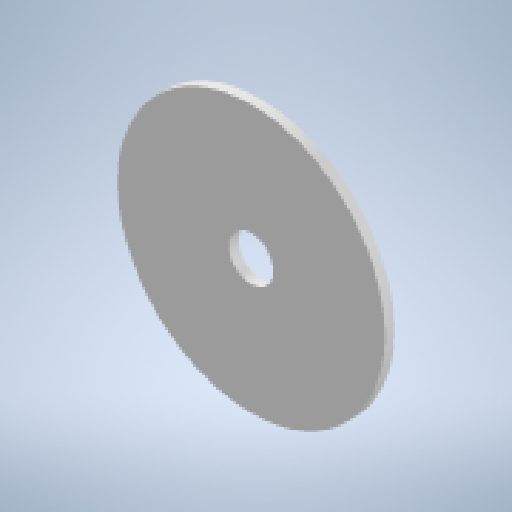
# Autodesk Inventor part: BaseTopPlate
Saved by Autodesk Inventor 2023 (Build 270158030, 158C)
## iProperties
Created: 2024-10-14
Part Number: BaseTopPlate
Material: Generic
Document SubType Name: Modeling
Designer: lvrectanus0
Density: 1 g/cm^3
Appearance: Default
Author: lvrectanus0
Autodesk Inventor part; units mm, degrees
ref_plane "YZ Plane" through (0, 0, 0) normal (1, 0, 0) x (0, 1, 0)
ref_plane "XZ Plane" through (0, 0, 0) normal (0, 1, 0) x (-1, 0, 0)
ref_plane "XY Plane" through (0, 0, 0) normal (0, 0, 1) x (1, 0, 0)
sketch "Sketch1" plane through (0, 0, 0) normal (0, 0, 1) x (1, 0, 0)
  circle A0 centre (0, 0) radius 14.2875 projected
  circle A1 centre (0, 0) radius 86.1483 projected
  point P0 (0, 0)
ref_plane "Work Plane1" through (-15.4305, -15.4305, -6.096) normal (0, 0, 1) x (1, 0, 0)
extrude "Extrusion1" add sketch "Sketch1" against normal up to surface (6.096 mm away)
sketch "Sketch2" plane through (0, 0, 0) normal (0, 0, 1) x (1, 0, 0)
  arc A0 (0.0676, -63.21) -> (-0.0676, -63.21) centre (0, -60.96) ccw projected
  circle A1 centre (0, -60.96) radius 3.175
  point P0 (0, 0)
  dimension "d2" = 6.35
  constraints: 1 centre point, 1 coincident
  measures "d2" diameter of A1
extrude "Extrusion2" cut sketch "Sketch2" against normal through all
chamfer "Chamfer1" distance 1 angle 45 2 edges at (-3.175, -60.96, -6.096) (-3.175, -60.96, 0)
sketch "Sketch3" plane through (0, 0, 0) normal (0, 0, 1) x (1, 0, 0)
  circle A0 centre (0, -60.96) radius 4.175 projected
  line L0 (15.5, -76.46) -> (-15.5, -45.46) construction
  line L1 (15.5, -45.46) -> (-15.5, -76.46) construction
  circle A1 centre (15.5, -76.46) radius 4
  circle A2 centre (-15.5, -76.46) radius 4
  circle A3 centre (-15.5, -45.46) radius 4
  circle A4 centre (15.5, -45.46) radius 4
  point P0 (0, 0)
  dimension "d8" = 31
  dimension "d9" = 31
  dimension "d10" = 8
  constraints: 4 centre point, 4 coincident, 4 end point, 3 equal radius, 2 horizontal alignment, 2 midpoint, 2 vertical alignment
  measures "d8" distance of L1.end L0.start
  measures "d9" distance of L0.end L1.end
  measures "d10" diameter of A1
sketch "Sketch4" plane through (0, 0, 0) normal (0, 0, 1) x (1, 0, 0)
  circle A0 centre (0, 0) radius 86.1483 projected
  circle A1 centre (0, -60.96) radius 3.175 projected
  circle A2 centre (50, 78.74) radius 2
  circle A3 centre (50, 27.94) radius 3
  circle A4 centre (50, 78.74) radius 7.1254
  circle A5 centre (0, 0) radius 86.1483 projected
  arc A6 (25.5581, 82.2698) -> (46.2963, 84.8272) centre (33.0936, 106.5263) ccw
  arc A7 (57.0844, 77.9767) -> (63.5895, 58.1198) centre (82.3382, 75.2559) ccw
  line L0 (0, 0) -> (0, 86.1483) construction
  circle A8 centre (-50, 78.74) radius 2
  circle A9 centre (-50, 27.94) radius 3
  circle A10 centre (-50, 78.74) radius 7.1254
  arc A11 (-46.2963, 84.8272) -> (-25.5581, 82.2698) centre (-33.0936, 106.5263) ccw
  arc A12 (-63.5895, 58.1198) -> (-57.0844, 77.9767) centre (-82.3382, 75.2559) ccw
  point P0 (0, 0)
  dimension "d25" = 60.96
  dimension "d36" = 4
  dimension "d37" = 6
  dimension "d38" = 50.8
  dimension "d39" = 50
  dimension "d40" = 27.94
  dimension "d42" = 25.4
  dimension "d43" = 25.4
  constraints: 15 point on circle, 10 centre point, 8 symmetric about line, 5 tangent, 2 end point, 1 vertical, 1 vertical alignment, 5 other
  measures "d25" distance of A1.centre point (0, 0)
  measures "d36" diameter of A2
  measures "d37" diameter of A3
  measures "d38" distance of A3.centre A2.centre
  measures "d39" horizontal distance of point (0, 0) A3.centre
  measures "d40" vertical distance of A3.centre point (0, 0)
  measures "d42" radius of A6
  measures "d43" radius of A7
extrude "Extrusion3" add sketch "Sketch3" along normal blind 5.08 contours A1 | A2 | A3 | A4
chamfer "Chamfer2" distance 1 angle 45 4 edges at (11.5, -45.46, 0) (11.5, -76.46, 0) (-19.5, -76.46, 0) (-19.5, -45.46, 0)
sketch "Sketch5" plane through (15.5, -76.46, 5.08) normal (0, 0, 1) x (1, 0, 0)
  circle A0 centre (0, 0) radius 4 projected
  circle A1 centre (-31, 0) radius 4 projected
  circle A2 centre (-31, 31) radius 4 projected
  circle A3 centre (0, 31) radius 4 projected
  point P0 (-15.5, 76.46)
hole "Hole1" at (15.5, -76.46, 5.08) at (-15.5, -76.46, 5.08) at (-15.5, -45.46, 5.08) at (15.5, -45.46, 5.08) direction (0, 0, -1) diameter 3.5 end through all
extrude "Extrusion4" add sketch "Sketch4" against normal up to surface (6.096 mm away) contours A0 A4 A7 | A12 A10 A0 | A0 A6 A4 | A4 | A10 A11 A0 | A10 | A2 | A8
hole "Hole2" at (-50, 78.74, 0) at (-50, 27.94, 0) at (50, 27.94, 0) at (50, 78.74, 0) direction (0, 0, -1) diameter 4 end through all
sketch "Sketch6" plane through (0, 0, 0) normal (0, 0, 1) x (1, 0, 0)
  line L0 (0, 0) -> (0, -12.7) construction
  line L1 (31.75, -12.7) -> (81.75, -12.7)
  line L2 (81.75, -12.7) -> (81.75, -6.35)
  line L3 (81.75, -6.35) -> (31.75, -6.35)
  line L4 (31.75, -6.35) -> (31.75, -12.7)
  dimension "d53" = 12.7
  dimension "d54" = 50
  dimension "d55" = 6.35
  dimension "d56" = 31.75
  constraints: 10 end point, 2 parallel, 1 horizontal, 1 horizontal alignment, 1 perpendicular, 1 vertical
  measures "d53" distance of L0.start L0.end
  measures "d54" distance of L3.end L2.end
  measures "d55" distance of L2.end L1.end
  measures "d56" horizontal distance of L0.start L3.end
extrude "Extrusion5" add sketch "Sketch6" along normal blind 50
fillet "Fillet1" radius 10 2 edges at (31.75, -9.525, 50) (81.75, -9.525, 50)
sketch "Sketch7" plane through (41.75, -12.7, 50) normal (0, -1, 0) x (1, 0, 0)
  line L0 (-0.5, -9.5) -> (30.5, -9.5)
  line L1 (30.5, -9.5) -> (30.5, -40.5)
  line L2 (30.5, -40.5) -> (-0.5, -40.5)
  line L3 (-0.5, -40.5) -> (-0.5, -9.5)
  arc A0 (40, -10) -> (30, 0) centre (30, -10) ccw construction
  arc A1 (0, 0) -> (-10, -10) centre (0, -10) ccw construction
  line L4 (30.5, -9.5) -> (-0.5, -40.5) construction
  line L5 (30.5, -40.5) -> (-0.5, -9.5) construction
  point P0 (-41.75, -50)
  point P1 (15, -25)
  point P2 (15, -25)
  dimension "d63" = 31
  dimension "d64" = 31
  constraints: 12 end point, 2 parallel, 2 point on line, 1 coincident, 1 horizontal, 1 midpoint, 1 perpendicular
  measures "d63" distance of L0.start L0.end
  measures "d64" distance of L0.end L1.end
hole "Hole3" at (41.75, -12.7, 40) at (72.25, -12.7, 40.5) at (41.25, -12.7, 9.5) at (72.25, -12.7, 9.5) direction (0, 1, 0) diameter 3.5 end through all
hole "Hole4" at (56.75, -12.7, 25) direction (0, 1, 0) diameter 6 end through all
sketch "Sketch8" plane through (31.75, -6.35, 0) normal (0, 1, 0) x (1, 0, 0)
  line L0 (0, 0) -> (0, -40) projected
  line L1 (0, 0) -> (2.54, 0)
  line L2 (2.54, 0) -> (2.54, -12.7)
  line L3 (2.54, -12.7) -> (0, -12.7)
  line L4 (0, -12.7) -> (0, 0)
  line L5 (50, 0) -> (0, 0) projected
  line L6 (25, 0) -> (22.46, 0)
  line L7 (22.46, 0) -> (22.46, -12.7)
  line L8 (22.46, -12.7) -> (25, -12.7)
  line L9 (25, -12.7) -> (25, 0)
  line L10 (50, 0) -> (47.46, 0)
  line L11 (47.46, 0) -> (47.46, -12.7)
  line L12 (47.46, -12.7) -> (50, -12.7)
  line L13 (50, -12.7) -> (50, 0)
  line L14 (25, 0) -> (27.54, 0)
  line L15 (27.54, 0) -> (27.54, -12.7)
  line L16 (27.54, -12.7) -> (25, -12.7)
  point P0 (-31.75, 0)
  point P1 (22.46, 0)
  dimension "d79" = 2.54
  dimension "d80" = 12.7
  dimension "d81" = 2.54
  dimension "d82" = 12.7
  constraints: 30 end point, 5 symmetric about line, 4 parallel, 2 horizontal, 2 perpendicular, 1 midpoint
  measures "d79" distance of L2.end L3.end
  measures "d80" distance of L1.end L2.end
  measures "d81" distance of L8.end L7.end
  measures "d82" distance of L7.end L6.end
extrude "Extrusion6" add sketch "Sketch8" along normal blind 12.7
chamfer "Chamfer4" distance 12.7 angle 45 3 edges at (80.48, 6.35, 12.7) (56.75, 6.35, 12.7) (33.02, 6.35, 12.7)
chamfer "Chamfer5" distance 3 angle 45 14 edges at (69.25, -6.35, 0) (44.25, -6.35, 0) (31.75, 6.35, 0) (31.75, -3.175, 0) (79.21, 0, 0) (79.21, 6.35, 0) (59.29, 0, 0) (59.29, 6.35, 0) (34.29, 6.35, 0) (34.29, 0, 0) (54.21, 0, 0) (54.21, 6.35, 0) (81.75, -3.175, 0) (81.75, 6.35, 0)
chamfer "Chamfer6" distance 1 angle 45 2 edges at (56.75, -12.7, 28) (56.75, -6.35, 28)
sketch "Sketch9" plane through (0, 0, -6.096) normal (0, 0, -1) x (-1, 0, 0)
  circle A0 centre (15.5, -76.46) radius 1.75 projected
  circle A1 centre (15.5, -45.46) radius 1.75 projected
  circle A2 centre (-15.5, -45.46) radius 1.75 projected
  circle A3 centre (-15.5, -76.46) radius 1.75 projected
  point P0 (0, 0)
  constraints: 4 coincident
hole "Hole5" at (-15.5, -76.46, -6.096) at (-15.5, -45.46, -6.096) at (15.5, -45.46, -6.096) at (15.5, -76.46, -6.096) direction (0, 0, 1) diameter 5 depth 4 tip angle 118
sketch "Sketch10" plane through (41.75, -6.35, 50) normal (0, 1, 0) x (1, 0, 0)
  circle A0 centre (0, 10) radius 1.75 projected
  circle A1 centre (-0.5, 40.5) radius 1.75 projected
  circle A2 centre (30.5, 40.5) radius 1.75 projected
  circle A3 centre (30.5, 9.5) radius 1.75 projected
  point P0 (-41.75, 50)
  constraints: 4 coincident
hole "Hole6" at (41.75, -6.35, 40) at (41.25, -6.35, 9.5) at (72.25, -6.35, 9.5) at (72.25, -6.35, 40.5) direction (0, -1, 0) diameter 5 depth 4 tip angle 118
sketch "Sketch11" plane through (0, 0, 0) normal (0, 0, 1) x (1, 0, 0)
  line L0 (-46.9642, -58.16) -> (-46.9642, -32.76)
  line L1 (-46.9642, -32.76) -> (-34.2642, -32.76)
  line L2 (-34.2642, -32.76) -> (-34.2642, -58.16)
  line L3 (-34.2642, -58.16) -> (-46.9642, -58.16)
  line L4 (-46.9642, -58.16) -> (-34.2642, -32.76) construction
  line L5 (-46.9642, -32.76) -> (-34.2642, -58.16) construction
  line L6 (-46.9642, -58.16) -> (-21.5642, -58.16) construction
  circle A0 centre (0, -60.96) radius 4.175 projected
  circle A1 centre (0, 0) radius 60.96
  circle A2 centre (-15.5, -45.46) radius 5 projected
  line L7 (-46.9642, -45.46) -> (-40.6142, -45.46)
  line L8 (-46.9642, -45.46) -> (-46.9642, -42.92)
  line L9 (-46.9642, -42.92) -> (-44.4242, -42.92)
  line L10 (-44.4242, -42.92) -> (-44.4242, -40.38)
  line L11 (-44.4242, -40.38) -> (-36.8042, -40.38)
  line L12 (-36.8042, -40.38) -> (-36.8042, -50.54)
  line L13 (-36.8042, -50.54) -> (-44.4242, -50.54)
  line L14 (-44.4242, -50.54) -> (-44.4242, -48)
  line L15 (-44.4242, -48) -> (-46.9642, -48)
  line L16 (-46.9642, -45.46) -> (-46.9642, -48)
  point P0 (-40.6142, -45.46)
  point P1 (-40.6142, -45.46)
  dimension "d108" = 25.4
  dimension "d109" = 90
  dimension "d110" = 12.7
  dimension "d111" = 2.54
  dimension "d112" = 2.54
  dimension "d113" = 2.54
  dimension "d114" = 7.62
  dimension "d115" = 10.16
  dimension "d116" = 7.62
  dimension "d117" = 2.54
  constraints: 34 end point, 8 perpendicular, 5 midpoint, 4 point on line, 2 parallel, 2 point on circle, 1 centre point, 1 coincident, 1 horizontal, 1 horizontal alignment
  measures "d108" distance of L0.start L0.end
  measures "d109" angle of L6 L0
  measures "d110" distance of L0.end L1.end
  measures "d111" distance of L7.start L8.end
  measures "d112" distance of L8.end L9.end
  measures "d113" distance of L9.end L10.end
  measures "d114" distance of L10.end L11.end
  measures "d115" distance of L11.end L12.end
  measures "d116" distance of L12.end L13.end
  measures "d117" distance of L13.end L14.end
extrude "Extrusion7" add sketch "Sketch11" along normal up to surface (50 mm away) contours L0 L15 L14 L13 L12 A1 L2 L3 | A1 L12 L11 L10 L0 L1 L2 | L0 A1 L10 L9
chamfer "Chamfer7" distance 1 angle 45 7 edges at (-40.6142, -40.38, 50) (-36.8042, -45.46, 50) (-40.6142, -50.54, 50) (-44.4242, -49.27, 50) (-44.4242, -41.65, 50) (-45.6942, -48, 50) (-45.6942, -42.92, 50)
chamfer "Chamfer8" distance 3 angle 45 3 edges at (-40.6142, -58.16, 0) (-34.2642, -45.46, 0) (-40.6142, -32.76, 0)
sketch "Sketch12" plane through (-46.9642, -58.16, 50) normal (0, -1, 0) x (1, 0, 0)
  line L0 (6.35, -6.35) -> (6.35, -38.1) construction
  line L1 (4.6, -6.35) -> (4.6, -38.1)
  line L2 (8.1, -38.1) -> (8.1, -6.35)
  arc A0 (8.1, -6.35) -> (4.6, -6.35) centre (6.35, -6.35) ccw
  arc A1 (4.6, -38.1) -> (8.1, -38.1) centre (6.35, -38.1) ccw
  line L3 (0, 0) -> (12.7, 0) construction
  line L4 (12.7, 0) -> (0, -12.7) construction
  line L5 (0, -50) -> (0, -1) construction
  line L6 (12.7, 0) -> (30.6605, 0) construction
  line L7 (0, 0) -> (12.7, -12.7) construction
  line L8 (12.7, -47) -> (12.7, 0) construction
  point P0 (46.9642, -50)
  point P1 (6.35, -22.225)
  dimension "d126" = 31.75
  dimension "d127" = 3.5
  dimension "d128" = 135
  constraints: 14 end point, 4 point on circle, 4 tangent, 2 centre point, 2 midpoint, 2 point on line, 1 equal length, 1 horizontal, 1 parallel, 1 vertical
  measures "d126" distance of L0.start L0.end
  measures "d127" diameter of A1
  measures "d128" angle of L4 L6
extrude "Extrusion8" cut sketch "Sketch12" against normal through all
chamfer "Chamfer9" distance 1 angle 45 23 edges at (-46.9642, -32.76, 26.5) (-34.2642, -32.76, 26.5) (-34.2642, -58.16, 26.5) (-46.9642, -58.16, 26.5) (-40.6142, -32.76, 50) (-34.2642, -45.46, 50) (-40.6142, -58.16, 50) (-40.6142, -58.16, 10.15) (-42.3642, -58.16, 27.775) (-40.6142, -58.16, 45.4) (-38.8642, -58.16, 27.775) (-40.6142, -32.76, 45.4) (-42.3642, -32.76, 27.775) (-40.6142, -32.76, 10.15) (-38.8642, -32.76, 27.775) (-40.6142, -40.38, 10.15) (-42.3642, -40.38, 27.775) (-40.6142, -40.38, 45.4) (-38.8642, -40.38, 27.775) (-40.6142, -50.54, 10.15) (-38.8642, -50.54, 27.775) (-40.6142, -50.54, 45.4) (-42.3642, -50.54, 27.775)
sketch "Sketch13" plane through (0, 0, 0) normal (0, 0, 1) x (1, 0, 0)
  circle A0 centre (50, 27.94) radius 2 projected
  circle A1 centre (-50, 78.74) radius 2 projected
  circle A2 centre (-50, 27.94) radius 2 projected
  circle A3 centre (50, 78.74) radius 2 projected
  circle A4 centre (-15.5, -76.46) radius 5 projected
  circle A5 centre (15.5, -45.46) radius 5 projected
  circle A6 centre (0, 0) radius 14.2875 projected
  arc A7 (-63.5895, 58.1198) -> (63.5895, 58.1198) centre (0, 0) ccw projected
  arc A8 (57.0844, 77.9767) -> (63.5895, 58.1198) centre (82.3382, 75.2559) ccw projected
  arc A9 (57.0844, 77.9767) -> (46.2963, 84.8272) centre (50, 78.74) ccw projected
  arc A10 (25.5581, 82.2698) -> (46.2963, 84.8272) centre (33.0936, 106.5263) ccw projected
  arc A11 (25.5581, 82.2698) -> (-25.5581, 82.2698) centre (0, 0) ccw projected
  arc A12 (-46.2963, 84.8272) -> (-25.5581, 82.2698) centre (-33.0936, 106.5263) ccw projected
  arc A13 (-46.2963, 84.8272) -> (-57.0844, 77.9767) centre (-50, 78.74) ccw projected
  arc A14 (-63.5895, 58.1198) -> (-57.0844, 77.9767) centre (-82.3382, 75.2559) ccw projected
  circle A15 centre (0, -60.96) radius 4.175 projected
  circle A16 centre (15.5, -76.46) radius 5 projected
  circle A17 centre (-15.5, -45.46) radius 5 projected
  line L0 (84.75, -12.7) -> (28.75, -12.7) projected
  line L1 (28.75, 6.35) -> (28.75, -12.7) projected
  line L2 (28.75, 6.35) -> (37.29, 6.35) projected
  line L3 (37.29, -3.35) -> (37.29, 6.35) projected
  line L4 (51.21, -3.35) -> (37.29, -3.35) projected
  line L5 (51.21, 6.35) -> (51.21, -3.35) projected
  line L6 (51.21, 6.35) -> (62.29, 6.35) projected
  line L7 (62.29, -3.35) -> (62.29, 6.35) projected
  line L8 (76.21, -3.35) -> (62.29, -3.35) projected
  line L9 (76.21, 6.35) -> (76.21, -3.35) projected
  line L10 (76.21, 6.35) -> (84.75, 6.35) projected
  line L11 (84.75, -12.7) -> (84.75, 6.35) projected
  line L12 (-46.9642, -42.92) -> (-46.9642, -29.76) projected
  line L13 (-31.2642, -29.76) -> (-46.9642, -29.76) projected
  line L14 (-31.2642, -61.16) -> (-31.2642, -29.76) projected
  line L15 (-46.9642, -61.16) -> (-31.2642, -61.16) projected
  line L16 (-46.9642, -61.16) -> (-46.9642, -48) projected
  line L17 (-46.9642, -48) -> (-44.4242, -48) projected
  line L18 (-44.4242, -48) -> (-44.4242, -50.54) projected
  line L19 (-44.4242, -50.54) -> (-36.8042, -50.54) projected
  line L20 (-36.8042, -50.54) -> (-36.8042, -40.38) projected
  line L21 (-36.8042, -40.38) -> (-44.4242, -40.38) projected
  line L22 (-44.4242, -40.38) -> (-44.4242, -42.92) projected
  line L23 (-44.4242, -42.92) -> (-46.9642, -42.92) projected
  circle A18 centre (0, 0) radius 19.3675
  circle A19 centre (-50, 27.94) radius 7.08
  circle A20 centre (50, 27.94) radius 7.08
  line L24 (39.195, 11.43) -> (26.845, 11.43)
  line L25 (23.67, 8.255) -> (23.67, -14.605)
  line L26 (26.845, -17.78) -> (89.83, -17.78)
  line L27 (89.83, -17.78) -> (89.83, 11.43)
  line L28 (76.5119, 11.43) -> (74.305, 11.43)
  line L29 (71.13, 8.255) -> (71.13, 1.73)
  line L30 (71.13, 1.73) -> (67.37, 1.73)
  line L31 (67.37, 1.73) -> (67.37, 8.255)
  line L32 (64.195, 11.43) -> (49.305, 11.43)
  line L33 (46.13, 8.255) -> (46.13, 1.73)
  line L34 (46.13, 1.73) -> (42.37, 1.73)
  line L35 (42.37, 1.73) -> (42.37, 8.255)
  circle A21 centre (15.5, -45.46) radius 10.08
  circle A22 centre (-15.5, -45.46) radius 10.08
  circle A23 centre (0, -60.96) radius 9.255
  circle A24 centre (-15.5, -76.46) radius 10.08
  circle A25 centre (15.5, -76.46) radius 10.08
  line L36 (-29.3592, -24.68) -> (-48.8692, -24.68)
  line L37 (-52.0442, -27.855) -> (-52.0442, -48)
  line L38 (-52.0442, -48) -> (-39.3442, -48)
  line L39 (-39.3442, -48) -> (-39.3442, -45.46)
  line L40 (-39.3442, -45.46) -> (-39.3442, -42.92)
  line L41 (-39.3442, -42.92) -> (-52.0442, -42.92)
  line L42 (-52.0442, -42.92) -> (-52.0442, -66.24)
  line L43 (-52.0442, -66.24) -> (-29.3592, -66.24)
  line L44 (-26.1842, -63.065) -> (-26.1842, -27.855)
  circle A26 centre (-50, 78.74) radius 7.08
  circle A27 centre (50, 78.74) radius 7.08
  arc A28 (79.6306, 15.2003) -> (59.8397, 54.6926) centre (0, 0) ccw
  arc A29 (-59.8397, 54.6926) -> (-52.0336, 78.5209) centre (-82.3382, 75.2559) ccw
  arc A30 (-48.9368, 80.4874) -> (-52.0336, 78.5209) centre (-50, 78.74) ccw
  arc A31 (-48.9368, 80.4874) -> (-24.051, 77.4185) centre (-33.0936, 106.5263) ccw
  arc A32 (24.051, 77.4185) -> (-24.051, 77.4185) centre (0, 0) ccw
  arc A33 (24.051, 77.4185) -> (48.9368, 80.4874) centre (33.0936, 106.5263) ccw
  arc A34 (52.0336, 78.5209) -> (48.9368, 80.4874) centre (50, 78.74) ccw
  arc A35 (52.0336, 78.5209) -> (59.8397, 54.6926) centre (82.3382, 75.2559) ccw
  line L45 (-19.6546, -48.242) -> (-7.6901, -66.1095)
  line L46 (-12.718, -41.3054) -> (5.1495, -53.2699)
  line L47 (12.718, -41.3054) -> (-5.1495, -53.2699)
  line L48 (19.6546, -48.242) -> (7.6901, -66.1095)
  line L49 (19.6546, -73.678) -> (7.6901, -55.8105)
  line L50 (-12.718, -80.6146) -> (5.1495, -68.6501)
  line L51 (-19.6546, -73.678) -> (-7.6901, -55.8105)
  line L52 (12.718, -80.6146) -> (-5.1495, -68.6501)
  line L53 (-20.4324, -44.6406) -> (-25.4437, -74.8082)
  line L54 (-25.4437, -47.1118) -> (-20.4324, -77.2794)
  line L55 (20.4324, -77.2794) -> (25.4437, -47.1118)
  line L56 (20.4324, -44.6406) -> (25.4437, -74.8082)
  line L57 (-16.3194, -40.5276) -> (13.8482, -35.5163)
  line L58 (16.3194, -40.5276) -> (-13.8482, -35.5163)
  circle A36 centre (-50, 78.74) radius 2 projected
  line L59 (-49.0942, 80.5231) -> (50.9058, 29.7231)
  circle A37 centre (50, 27.94) radius 2 projected
  line L60 (49.0942, 26.1569) -> (-50.9058, 76.9569)
  circle A38 centre (-50, 27.94) radius 2 projected
  line L61 (-50.9058, 29.7231) -> (49.0942, 80.5231)
  circle A39 centre (50, 78.74) radius 2 projected
  line L62 (-49.0942, 26.1569) -> (50.9058, 76.9569)
  circle A40 centre (-50, 27.94) radius 2
  circle A41 centre (50, 78.74) radius 2
  circle A42 centre (50, 27.94) radius 2
  circle A43 centre (-50, 78.74) radius 2
  arc A44 (48.0344, 21.1383) -> (-48.0344, 21.1383) centre (0, -145.0737) ccw
  arc A45 (56.0591, 75.0776) -> (56.0591, 31.6024) centre (92.0221, 53.34) ccw
  arc A46 (49.4447, 26.0186) -> (-49.4447, 26.0186) centre (0, -145.0737) ccw
  arc A47 (51.7116, 77.7054) -> (51.7116, 28.9746) centre (92.0221, 53.34) ccw
  arc A48 (-56.0591, 31.6024) -> (-56.0591, 75.0776) centre (-92.0221, 53.34) ccw
  arc A49 (-51.7116, 28.9746) -> (-51.7116, 77.7054) centre (-92.0221, 53.34) ccw
  arc A50 (-45.9629, 33.7562) -> (0, 19.3675) centre (0, 99.9732) ccw
  arc A51 (-19.3675, 0) -> (-47.9379, 21.1669) centre (-41.4937, 0) ccw
  arc A52 (0, 19.3675) -> (45.9629, 33.7562) centre (0, 99.9732) ccw
  arc A53 (47.9379, 21.1669) -> (19.3675, 0) centre (41.4937, 0) ccw
  arc A54 (26.845, 11.43) -> (23.67, 8.255) centre (26.845, 8.255) ccw
  arc A55 (42.37, 8.255) -> (39.195, 11.43) centre (39.195, 8.255) ccw
  arc A56 (49.305, 11.43) -> (46.13, 8.255) centre (49.305, 8.255) ccw
  arc A57 (67.37, 8.255) -> (64.195, 11.43) centre (64.195, 8.255) ccw
  arc A58 (74.305, 11.43) -> (71.13, 8.255) centre (74.305, 8.255) ccw
  arc A59 (76.5119, 11.43) -> (79.6306, 15.2003) centre (76.5119, 14.605) ccw
  arc A60 (23.67, -14.605) -> (26.845, -17.78) centre (26.845, -14.605) ccw
  arc A61 (-63.5895, 58.1198) -> (63.5895, 58.1198) centre (0, 0) ccw projected
  circle A62 centre (0, 0) radius 81.0683
  circle A63 centre (-86.1483, 0) radius 14.2875
  arc A64 (-80.0333, 12.9128) -> (-6.115, 12.9128) centre (-43.0742, 90.9578) ccw
  circle A65 centre (0, 0) radius 14.2875 projected
  arc A66 (-6.115, -12.9128) -> (-80.0333, -12.9128) centre (-43.0742, -90.9578) ccw
  arc A67 (-48.0344, 21.1383) -> (-72.3431, -3.6807) centre (-38.2336, -12.7748) ccw
  arc A68 (-86.3236, 14.2864) -> (-56.0591, 31.6024) centre (-86.7639, 50.1617) ccw
  circle A69 centre (86.1483, 0) radius 14.2875
  arc A70 (6.115, 12.9128) -> (80.0333, 12.9128) centre (43.0742, 90.9578) ccw
  arc A71 (80.0333, -12.9128) -> (10.0594, -16.5502) centre (48.4218, -79.6655) ccw
  arc A72 (-24.4083, -40.7432) -> (-14.2875, 0) centre (-101.3575, 0) ccw
  arc A73 (14.2875, 0) -> (24.4083, -40.7432) centre (101.3575, 0) ccw
  arc A74 (-48.8692, -24.68) -> (-52.0442, -27.855) centre (-48.8692, -27.855) ccw
  arc A75 (-26.1842, -27.855) -> (-29.3592, -24.68) centre (-29.3592, -27.855) ccw
  arc A76 (-29.3592, -66.24) -> (-26.1842, -63.065) centre (-29.3592, -63.065) ccw
  arc A77 (-39.1142, -24.68) -> (-14.2875, 0) centre (-39.1142, 0.1471) ccw
  arc A78 (-65.7994, -47.3552) -> (-52.0442, -42.92) centre (-59.6368, -42.92) ccw
  arc A79 (58.3375, -17.78) -> (25.5003, -46.725) centre (58.3375, -50.8789) ccw
  arc A80 (25.5003, -46.725) -> (52.891, -61.4379) centre (42.0244, -48.8153) ccw
  arc A81 (70.9696, -39.1841) -> (58.3375, -17.78) centre (58.3375, -32.2096) ccw
  arc A82 (72.3431, -3.6807) -> (48.0344, 21.1383) centre (38.2336, -12.7748) ccw
  arc A83 (56.0591, 31.6024) -> (86.3236, 14.2864) centre (86.7639, 50.1617) ccw
  point P0 (0, 0)
  point P1 (0, 27.94)
  point P2 (50, 53.34)
  point P3 (-50, 53.34)
  point P4 (23.1433, -60.96)
  point P5 (21.8667, -53.2748)
  point P6 (14.7847, -55.5146)
  point P7 (11.1383, -60.96)
  point P8 (14.7847, -66.4054)
  point P9 (21.8667, -68.6452)
  point P10 (-6.4091, -80.8146)
  point P11 (6.4091, -80.8146)
  point P12 (5.4454, -75.7447)
  point P13 (0, -72.0983)
  point P14 (-5.4454, -75.7447)
  point P15 (-23.1433, -60.96)
  point P16 (-21.8667, -68.6452)
  point P17 (-14.7847, -66.4054)
  point P18 (-11.1383, -60.96)
  point P19 (-14.7847, -55.5146)
  point P20 (-21.8667, -53.2748)
  point P21 (7.6852, -39.0933)
  point P22 (0, -37.8167)
  point P23 (-7.6852, -39.0933)
  point P24 (-5.4454, -46.1753)
  point P25 (0, -49.8217)
  point P26 (5.4454, -46.1753)
  point P27 (-16.5111, -10.1235)
  point P28 (-17.398, -8.5094)
  point P29 (-48.6812, 34.8961)
  point P30 (-44.6817, 32.885)
  point P31 (-4.4159, 53.34)
  point P32 (-44.8507, 73.8809)
  point P33 (-48.6812, 71.7839)
  point P34 (-48.0344, 21.1383)
  point P35 (-66.8224, 7.9335)
  point P36 (-20.6968, 7.5536)
  point P37 (-47.171, 21.3854)
  point P38 (30.2775, 25.2701)
  point P39 (-30.2775, 25.2701)
  point P40 (-79.67, 14.992)
  point P41 (-56.0591, 31.6024)
  point P42 (-52.6974, 68.153)
  point P43 (0, 55.5833)
  point P44 (43.039, 77.4471)
  point P45 (42.9968, 77.6999)
  point P46 (-42.9968, 77.6999)
  point P47 (-43.039, 77.4471)
  point P48 (38.0424, 28.9095)
  point P49 (40.7217, 30.4101)
  point P50 (0, 51.0967)
  point P51 (-40.7217, 30.4101)
  point P52 (-38.0424, 28.9095)
  point P53 (4.4159, 53.34)
  point P54 (44.6817, 32.885)
  point P55 (48.6812, 34.8961)
  point P56 (48.6812, 71.7839)
  point P57 (44.8507, 73.8809)
  point P58 (42.37, 4.6067)
  point P59 (46.13, 4.6579)
  point P60 (63.9296, 11.43)
  point P61 (48.0344, 21.1383)
  point P62 (47.171, 21.3854)
  point P63 (20.6968, 7.5536)
  point P64 (23.67, 6.8122)
  point P65 (56.0591, 31.6024)
  point P66 (79.663, 14.9934)
  point P67 (52.6974, 68.153)
  dimension "d144" = 5.08
  dimension "d145" = 5.08
  dimension "d134" = 5.08
  dimension "d135" = 5.08
  dimension "d136" = 5.08
  dimension "d137" = 5.08
  dimension "d138" = 5.08
  dimension "d139" = 5.08
  dimension "d140" = 5.08
  dimension "d141" = 5.08
  dimension "d142" = 5.08
  dimension "d143" = 5.08
  dimension "d146" = 5.08
  dimension "d147" = 3.175
  dimension "d148" = 3.175
  constraints: 143 point on circle, 78 end point, 77 tangent, 53 centre point, 8 equal radius, 7 horizontal alignment, 5 coincident, 3 perpendicular, 3 vertical alignment, 2 midpoint, 1 concentric, 1 point on line, 105 other
  measures "d136" radial gap between concentric circles of A0 A20
  measures "d137" distance between parallel lines of L2 L24
  measures "d138" radial gap between concentric circles of A5 A21
  measures "d139" radial gap between concentric circles of A17 A22
  measures "d143" distance between parallel lines of L14 L44
  measures "d146" radial gap between concentric circles of A7 A28
  measures "d147" radius of A54
  measures "d148" radius of A74
extrude "Extrusion9" cut sketch "Sketch13" against normal through all contours A20 A52 L59 L62 A62 A47 | A45 A62 A28 A59 A83 | A62 L62 A27 A47 | A20 A82 L32 A56 L33 A70 L35 A55 L24 A54 L25 A53 A44 | A46 A50 L62 L60 A52 | A45 A35 A62 | A52 A50 A44 | A62 A33 A27 L61 | L61 L59 A62 A32 | L61 A50 A19 A49 A62 L60 | A44 A51 A64 A67 A19 | L59 A26 A31 A62 | A62 A49 A26 L60 | A68 A62 A48 | A18 A77 L36 A74 L37 A78 A62 A66 | A62 A29 A48 | A81 A62 A80 A79 | A21 L47 L46 A22 L57 L58 | A62 A24 L50 L52 A25 | A22 L45 L51 A24 L54 L53 | L56 L55 A25 L49 L48 A21
body "Solid1"
